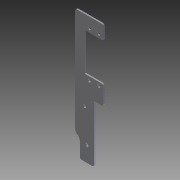
# Autodesk Inventor part: riset tibia alumunium 1
Saved by Autodesk Inventor 2012 (Build 160160000, 160)
## iProperties
Created: 2013-11-27
Part Number: riset tibia alumunium 1
Material: Default
Document SubType Name: Modeling
Designer: Irwan Haryanto
Density: 1 g/cm^3
Author: Irwan Haryanto
Autodesk Inventor part; units mm, degrees
ref_plane "YZ Plane" through (0, 0, 0) normal (1, 0, 0) x (0, 1, 0)
ref_plane "XZ Plane" through (0, 0, 0) normal (0, 1, 0) x (-1, 0, 0)
sketch "Sketch1" plane through (0, 0, 0) normal (0, 0, 1) x (1, 0, 0)
  line L0 (-13.9785, 19.8477) -> (4.0215, 19.8477)
  line L1 (4.0215, -20.1523) -> (-13.9785, -20.1523)
  line L2 (-13.9785, -20.1523) -> (-13.9785, 19.8477)
  line L3 (6.0215, -22.1523) -> (6.0215, -38.1523)
  line L4 (6.0215, 21.8477) -> (6.0215, 32.8477)
  circle A0 centre (-3.9785, -10.9023) radius 2.5
  line L5 (6.0215, 19.8477) -> (6.0215, 34.8477)
  line L6 (6.0215, -20.1523) -> (6.0215, -40.1523)
  line L7 (4.0215, -40.1523) -> (-1.9785, -40.1523)
  line L8 (-3.9785, -80.9023) -> (-3.9785, -95.9023)
  line L9 (-3.9785, -98.9023) -> (-3.9785, -42.1523)
  line L10 (-23.9785, 32.8477) -> (-23.9785, -75.9023)
  line L11 (6.0215, 19.8477) -> (6.0215, 34.8477)
  circle A1 centre (-8.9785, -24.1523) radius 1.5
  circle A2 centre (1.0215, -24.1523) radius 1.5
  circle A3 centre (-8.9785, 23.8477) radius 1.5
  circle A4 centre (1.0215, 23.8477) radius 1.5
  line L12 (-5.9785, -100.9023) -> (-16.9785, -100.9023)
  line L13 (6.0215, 19.8477) -> (6.0215, 21.4291)
  line L14 (6.0215, 19.8477) -> (6.0215, 34.8477)
  line L15 (4.0215, 34.8477) -> (-21.9785, 34.8477)
  line L16 (-18.9785, -98.9023) -> (-18.9785, -84.5626)
  line L17 (-18.9785, -80.9023) -> (-18.9785, -80.9023)
  arc A5 (-18.9785, -98.9023) -> (-16.9785, -100.9023) centre (-16.9785, -98.9023) ccw
  arc A6 (-5.9785, -100.9023) -> (-3.9785, -98.9023) centre (-5.9785, -98.9023) ccw
  arc A7 (-1.9785, -40.1523) -> (-3.9785, -42.1523) centre (-1.9785, -42.1523) ccw
  arc A8 (4.0215, -40.1523) -> (6.0215, -38.1523) centre (4.0215, -38.1523) ccw
  arc A9 (6.0215, -22.1523) -> (4.0215, -20.1523) centre (4.0215, -22.1523) ccw
  arc A10 (4.0215, 19.8477) -> (6.0215, 21.8477) centre (4.0215, 21.8477) ccw
  arc A11 (6.0215, 32.8477) -> (4.0215, 34.8477) centre (4.0215, 32.8477) ccw
  arc A12 (-21.9785, 34.8477) -> (-23.9785, 32.8477) centre (-21.9785, 32.8477) ccw
  arc A13 (-23.9785, -75.9023) -> (-21.4785, -80.2325) centre (-18.9785, -75.9023) ccw
  arc A14 (-18.9785, -84.5626) -> (-21.4785, -80.2325) centre (-23.9785, -84.5626) ccw
  circle A15 centre (-13.9785, -50.1523) radius 1.5
  circle A16 centre (-11.4785, -84.5626) radius 1.5
  point P0 (0, 0)
  point P1 (0, 0)
  point P2 (0, 0)
  point P3 (-23.9785, 34.8477)
  point P4 (-3.9785, -100.9023)
  point P5 (-18.9785, -100.9023)
  dimension "d0" = 5
  dimension "d1" = 20
  dimension "d2" = 3
  dimension "d3" = 5
  dimension "d4" = 4
  dimension "d5" = 3
  dimension "d6" = 10
  dimension "d7" = 3
  dimension "d8" = 3
  dimension "d9" = 10
  dimension "d10" = 5
  dimension "d11" = 4
  dimension "d14" = 15
  dimension "d15" = 135.75
  dimension "d18" = 10
  dimension "d19" = 15
  dimension "d21" = 30
  dimension "d22" = 2
  dimension "d23" = 5
  dimension "d26" = 3
  dimension "d27" = 3
  dimension "d29" = 30
  dimension "d62" = 48
  dimension "d63" = 48
  constraints: 36 end point, 21 point on circle, 20 tangent, 17 centre point, 17 point on line, 8 equal radius, 4 perpendicular, 2 equal length, 1 horizontal
  measures "d0" diameter of A0
  measures "d1" distance of L6.start L6.end
  measures "d2" diameter of A1
  measures "d3" distance from line of A1.centre L2
  measures "d4" distance from line of L1 A1.centre
  measures "d5" diameter of A2
  measures "d6" distance of A2.centre A1.centre
  measures "d7" diameter of A3
  measures "d8" diameter of A4
  measures "d9" distance of A4.centre A3.centre
  measures "d10" distance from line of A3.centre L2
  measures "d11" distance from line of L0 A3.centre
  measures "d14" distance of L5.start L5.end
  measures "d15" distance between parallel lines of L12 L15
  measures "d18" distance between parallel lines of L3 L9
  measures "d19" distance of point (-3.978, -100.902) point (-18.978, -100.902)
  measures "d21" distance of L5.end point (-23.978, 34.848)
  measures "d22" radius of A5
  measures "d23" radius of A13
  measures "d26" diameter of A15
  measures "d27" diameter of A16
  measures "d29" distance from line of A15.centre L1
  measures "d62" distance of A2.centre A4.centre
  measures "d63" distance of A1.centre A3.centre
extrude "Extrusion2" add sketch "Sketch1" along normal blind 1.5 contours L2 L1 A9 L3 A8 L7 A7 L9 L8 A6 L12 A5 L16 A14 A13 L10 A12 L15 A11 L4 A10 L0 | A1 | A2 | A3 | A4 | A15 | A16
ref_plane "Work Plane1" through (0, 0, 1.5) normal (0, 0, 1) x (1, 0, 0)
sketch "Sketch4" plane through (0, 0, 1.5) normal (0, 0, 1) x (1, 0, 0)
  line L0 (-13.9785, 19.8477) -> (4.0215, 19.8477)
  line L1 (4.0215, -20.1523) -> (-13.9785, -20.1523)
  line L2 (-13.9785, -20.1523) -> (-13.9785, 19.8477)
  line L3 (6.0215, -22.1523) -> (6.0215, -38.1523)
  line L4 (6.0215, 21.8477) -> (6.0215, 32.8477)
  circle A0 centre (-3.9785, -10.9023) radius 2.5
  line L5 (6.0215, 19.8477) -> (6.0215, 34.8477)
  line L6 (6.0215, -20.1523) -> (6.0215, -40.1523)
  line L7 (4.0215, -40.1523) -> (-1.9785, -40.1523)
  line L8 (-3.9785, -80.9023) -> (-3.9785, -95.9023)
  line L9 (-3.9785, -98.9023) -> (-3.9785, -42.1523)
  line L10 (-23.9785, 32.8477) -> (-23.9785, -75.9023)
  line L11 (6.0215, 19.8477) -> (6.0215, 34.8477)
  circle A1 centre (-8.9785, -24.1523) radius 1.5
  circle A2 centre (1.0215, -24.1523) radius 1.5
  circle A3 centre (-8.9785, 23.8477) radius 1.5
  circle A4 centre (1.0215, 23.8477) radius 1.5
  line L12 (-5.9785, -100.9023) -> (-16.9785, -100.9023)
  line L13 (6.0215, 19.8477) -> (6.0215, 21.4291)
  line L14 (6.0215, 19.8477) -> (6.0215, 34.8477)
  line L15 (4.0215, 34.8477) -> (-21.9785, 34.8477)
  line L16 (-18.9785, -98.9023) -> (-18.9785, -84.5626)
  line L17 (-18.9785, -80.9023) -> (-18.9785, -80.9023)
  arc A5 (-18.9785, -98.9023) -> (-16.9785, -100.9023) centre (-16.9785, -98.9023) ccw
  arc A6 (-5.9785, -100.9023) -> (-3.9785, -98.9023) centre (-5.9785, -98.9023) ccw
  arc A7 (-1.9785, -40.1523) -> (-3.9785, -42.1523) centre (-1.9785, -42.1523) ccw
  arc A8 (4.0215, -40.1523) -> (6.0215, -38.1523) centre (4.0215, -38.1523) ccw
  arc A9 (6.0215, -22.1523) -> (4.0215, -20.1523) centre (4.0215, -22.1523) ccw
  arc A10 (4.0215, 19.8477) -> (6.0215, 21.8477) centre (4.0215, 21.8477) ccw
  arc A11 (6.0215, 32.8477) -> (4.0215, 34.8477) centre (4.0215, 32.8477) ccw
  arc A12 (-21.9785, 34.8477) -> (-23.9785, 32.8477) centre (-21.9785, 32.8477) ccw
  arc A13 (-23.9785, -75.9023) -> (-21.4785, -80.2325) centre (-18.9785, -75.9023) ccw
  arc A14 (-18.9785, -84.5626) -> (-21.4785, -80.2325) centre (-23.9785, -84.5626) ccw
  circle A15 centre (-13.9785, -50.1523) radius 1.5
  circle A16 centre (-11.4785, -84.5626) radius 1.5
  point P0 (0, 0)
  point P1 (0, 0)
  point P2 (0, 0)
  point P3 (0, 0)
  point P4 (-23.9785, 34.8477)
  point P5 (-3.9785, -100.9023)
  point P6 (-18.9785, -100.9023)
  dimension "d33" = 5
  dimension "d34" = 20
  dimension "d35" = 3
  dimension "d36" = 5
  dimension "d37" = 4
  dimension "d38" = 3
  dimension "d39" = 10
  dimension "d40" = 3
  dimension "d41" = 3
  dimension "d42" = 10
  dimension "d43" = 5
  dimension "d44" = 4
  dimension "d45" = 15
  dimension "d46" = 135.75
  dimension "d47" = 10
  dimension "d48" = 15
  dimension "d49" = 30
  dimension "d50" = 2
  dimension "d51" = 5
  dimension "d52" = 3
  dimension "d53" = 3
  dimension "d54" = 30
  constraints: 36 end point, 21 point on circle, 20 tangent, 17 centre point, 17 point on line, 8 equal radius, 4 perpendicular, 2 equal length, 1 horizontal
  measures "d33" diameter of A0
  measures "d34" distance of L6.start L6.end
  measures "d35" diameter of A1
  measures "d36" distance from line of A1.centre L2
  measures "d37" distance from line of L1 A1.centre
  measures "d38" diameter of A2
  measures "d39" distance of A2.centre A1.centre
  measures "d40" diameter of A3
  measures "d41" diameter of A4
  measures "d42" distance of A4.centre A3.centre
  measures "d43" distance from line of A3.centre L2
  measures "d44" distance from line of L0 A3.centre
  measures "d45" distance of L5.start L5.end
  measures "d46" distance between parallel lines of L12 L15
  measures "d47" distance between parallel lines of L3 L9
  measures "d48" distance of point (-3.978, -100.902) point (-18.978, -100.902)
  measures "d49" distance of L5.end point (-23.978, 34.848)
  measures "d50" radius of A5
  measures "d51" radius of A13
  measures "d52" diameter of A15
  measures "d53" diameter of A16
  measures "d54" distance from line of A15.centre L1
hole "Hole1" at (-8.9785, 23.8477, 1.5) at (1.0215, 23.8477, 1.5) at (-8.9785, -24.1523, 1.5) at (1.0215, -24.1523, 1.5) at (-13.9785, -50.1523, 1.5) at (-11.4785, -84.5626, 1.5) direction (0, 0, -1) diameter 3 end through all
body "Solid2"
